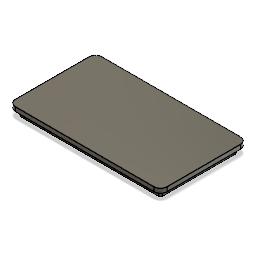
Sensor lid (Autodesk Fusion 360 design; units mm, degrees)
Autodesk Fusion 360 part; units mm, degrees
sketch "Sketch1" plane through (0, 0, 0) normal (0, 1, 0) x (1, 0, 0)
  line L0 (-35, 20) -> (35, 20)
  line L1 (35, 20) -> (35, -20)
  line L2 (35, -20) -> (-35, -20)
  line L3 (-35, -20) -> (-35, 20)
  line L4 (-35, 20) -> (35, -20) construction
  dimension "d106" = 70
  dimension "d107" = 40
  constraint horizontal L0
  constraint vertical L1
  constraint horizontal L2
  constraint vertical L3
  constraint midpoint origin L4
  measures "d106" distance of L0.start L0.end
  measures "d107" distance of L0.end L1.end
extrude "Extrude1" add sketch "Sketch1" along normal blind 2
fillet "Fillet1" radius 3 4 edges at (-35, 1, 20) (35, 1, -20) (-35, 1, -20) (35, 1, 20)
sketch "Sketch2" plane through (0, 0, 0) normal (0, -1, 0) x (1, 0, 0)
  arc A0 (35, 17) -> (32, 20) centre (32, 17) ccw
  line L0 (32, 20) -> (-32, 20)
  arc A1 (-32, 20) -> (-35, 17) centre (-32, 17) ccw
  line L1 (-35, 17) -> (-35, -17)
  arc A2 (-35, -17) -> (-32, -20) centre (-32, -17) ccw
  line L2 (-32, -20) -> (32, -20)
  arc A3 (32, -20) -> (35, -17) centre (32, -17) ccw
  line L3 (35, -17) -> (35, 17)
  line L4 (-32.8, 17) -> (-32.8, -17)
  arc A4 (-32.8, -17) -> (-32, -17.8) centre (-32, -17) ccw
  line L5 (-32, -17.8) -> (32, -17.8)
  arc A5 (32, -17.8) -> (32.8, -17) centre (32, -17) ccw
  line L6 (32.8, -17) -> (32.8, 17)
  arc A6 (32.8, 17) -> (32, 17.8) centre (32, 17) ccw
  line L7 (32, 17.8) -> (-32, 17.8)
  arc A7 (-32, 17.8) -> (-32.8, 17) centre (-32, 17) ccw
  line L8 (-31.8, 16.8) -> (-31.8, -16.8)
  line L9 (-31.8, -16.8) -> (31.8, -16.8)
  line L10 (31.8, -16.8) -> (31.8, 16.8)
  line L11 (31.8, 16.8) -> (-31.8, 16.8)
  dimension "d111" = -2.2
  dimension "d112" = -3.2
extrude "Extrude2" add sketch "Sketch2" along normal blind 3 contours L4 A4 L5 A5 L6 A6 L7 A7
